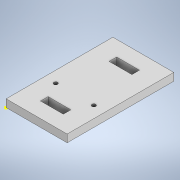
# Autodesk Inventor part: wrist_plate
Saved by Autodesk Inventor 2022 (Build 260153000, 153)
## iProperties
Created: 2022-01-26
Part Number: wrist_plate
Material: Generic
Document SubType Name: Modeling
Designer: pauly
Density: 1 g/cm^3
Appearance: Default
Author: pauly
Autodesk Inventor part; units mm, degrees
ref_plane "YZ Plane" through (0, 0, 0) normal (1, 0, 0) x (0, 1, 0)
ref_plane "XZ Plane" through (0, 0, 0) normal (0, 1, 0) x (-1, 0, 0)
ref_plane "XY Plane" through (0, 0, 0) normal (0, 0, 1) x (1, 0, 0)
sketch "Sketch1" plane through (0, 0, 0) normal (0, 1, 0) x (-1, 0, 0)
  point P0 (0, 0)
sketch "Sketch2" plane through (0, 0, 0) normal (0, 1, 0) x (-1, 0, 0)
  point P0 (0, 0)
sketch "Sketch3" plane through (0, 0, 0) normal (0, 1, 0) x (-1, 0, 0)
  point P0 (0, 0)
sketch "Sketch4" plane through (0, 0, 0) normal (0, 1, 0) x (-1, 0, 0)
  line L0 (0, 0) -> (-101.6, 0)
  line L1 (-101.6, 0) -> (-101.6, -177.8)
  line L2 (-101.6, -177.8) -> (0, -177.8)
  line L3 (0, -177.8) -> (0, 0)
  line L4 (-50.8, -25.4) -> (-69.85, -25.4)
  line L5 (-69.85, -25.4) -> (-31.75, -25.4)
  line L6 (-31.75, -25.4) -> (-31.75, -38.1)
  line L7 (-31.75, -38.1) -> (-69.85, -38.1)
  line L8 (-69.85, -38.1) -> (-69.85, -25.4)
  line L9 (-50.8, -177.8) -> (-50.8, -152.4)
  line L10 (-50.8, -152.4) -> (-31.75, -152.4)
  line L11 (-31.75, -152.4) -> (-31.75, -139.7)
  line L12 (-31.75, -139.7) -> (-69.85, -139.7)
  line L13 (-69.85, -139.7) -> (-69.85, -152.4)
  line L14 (-69.85, -152.4) -> (-50.8, -152.4)
  dimension "d0" = 101.6
  dimension "d1" = 177.8
  dimension "d3" = 19.05
  dimension "d4" = 38.1
  dimension "d5" = 12.7
  dimension "d6" = 38.1
  dimension "d7" = 25.4
  dimension "d8" = 19.05
  dimension "d9" = 12.7
  dimension "d10" = 38.1
  dimension "d11" = 12.7
  constraints: 30 end point, 7 perpendicular, 2 parallel, 2 point on line, 1 horizontal, 1 midpoint, 1 vertical
  measures "d0" distance of L2.end L1.end
  measures "d1" distance of L0.end L1.end
  measures "d3" distance of L4.start L4.end
  measures "d4" distance of L4.end L5.end
  measures "d5" distance of L5.end L6.end
  measures "d6" distance of L6.end L7.end
  measures "d7" distance of L9.start L9.end
  measures "d8" distance of L9.end L10.end
  measures "d9" distance of L10.end L11.end
  measures "d10" distance of L11.end L12.end
  measures "d11" distance of L12.end L13.end
extrude "Extrusion1" add sketch "Sketch4" along normal blind 12.7
sketch "Sketch5" plane through (0, 12.7, 0) normal (0, 1, 0) x (1, 0, 0)
  circle A0 centre (19.05, 63.5) radius 3.9688
  circle A1 centre (82.55, 63.5) radius 3.9687
  point P0 (0, 0)
  point P1 (31.75, 38.1)
  dimension "d19" = 7.9375
  dimension "d21" = 7.9375
  constraints: 2 centre point
  measures "d19" diameter of A0
  measures "d21" diameter of A1
hole "Hole1" at (19.05, 12.7, -63.5) direction (0, -1, 0) diameter 6.4008 end through all thread size "5/16-18 UNC" class "2B" standard "ANSI Unified Screw Threads"
hole "Hole2" at (82.55, 12.7, -63.5) direction (0, -1, 0) diameter 6.4008 end through all thread size "5/16-18 UNC" class "2B" standard "ANSI Unified Screw Threads"
equation "\"d23\" = d12"
equation "\"d30\" = d12"
equation "\"d12\" = 12.7"
body "Solid1"
